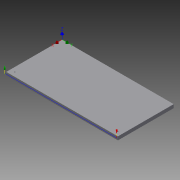
# Autodesk Inventor part: placa 12mm suport electronica
Saved by Autodesk Inventor 2015 SP1 (Build 190203100, 203)
## iProperties
Created: 2015-05-04
Part Number: placa 12mm suport electronica
Material: Generic
Document SubType Name: Modeling
Designer: ubik
Density: 1 g/cm^3
Appearance: Default
Author: ubik
Autodesk Inventor part; units mm, degrees
ref_plane "YZ Plane" through (0, 0, 0) normal (1, 0, 0) x (0, 1, 0)
ref_plane "XZ Plane" through (0, 0, 0) normal (0, 1, 0) x (-1, 0, 0)
ref_plane "XY Plane" through (0, 0, 0) normal (0, 0, 1) x (1, 0, 0)
sketch "Sketch1" plane through (0, 0, 0) normal (0, 0, 1) x (1, 0, 0)
  line L0 (0, 0) -> (390, 0)
  line L1 (390, 0) -> (390, 195)
  line L2 (390, 195) -> (0, 195)
  line L3 (0, 195) -> (0, 0)
  dimension "d0" = 390
  dimension "d1" = 195
  constraints: 8 end point, 2 parallel, 1 horizontal, 1 perpendicular
  measures "d0" distance of L1.end L2.end
  measures "d1" distance of L0.end L1.end
extrude "Extrusion1" add sketch "Sketch1" along normal blind 12
hole "Hole1" at (15, 15, 12) direction (0, 0, -1) diameter 3 end through all
pattern_linear "Rectangular Pattern1" count 2 spacing 200 along (0, 1, 0) count 2 spacing 360 along (1, 0, 0) of "Hole1"
body "Solid1"
